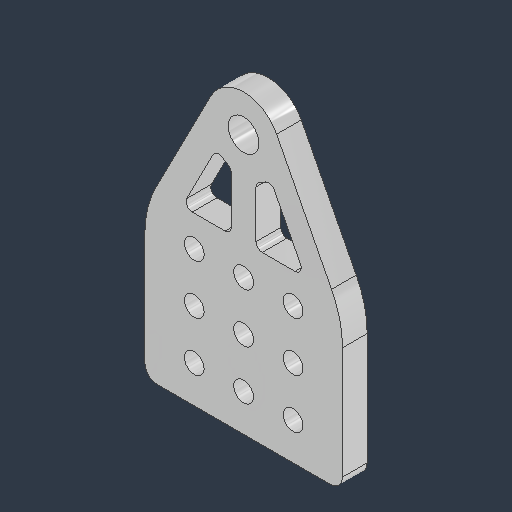
# Autodesk Inventor part: PLATE,SIDE,PULLEY,MOUNT,TOP,ELEVATORR
Saved by Autodesk Inventor 2024.3 (Build 283343000, 343)
## iProperties
ILogicPurgeVersion: 0.0.0.0
OnSaveVersion: 3.4.3.0
OnSaveAssembly: COREAutomationManager
Created: 2025-01-27
Part Number: PLATE,SIDE,PULLEY,MOUNT,TOP,ELEVATORR
Material: Aluminum 7075
Document SubType Name: Modeling
Designer: Jthib
Density: 2.81 g/cm^3
Appearance: Aluminum - Polished
Mfg Approved By: John.Thibert
Sheet Metal Rule: Default
Mass: 83.4067 g
Surface Area: 97.3008 cm^2
Volume: 29.6821 cm^3
ModelCat: Uncategorized
MaterialName: Aluminum 7075
CN_MASS: 0.08
Author: Jthib
Autodesk Inventor part; units mm, degrees
ref_plane "YZ Plane" through (0, 0, 0) normal (1, 0, 0) x (0, 1, 0)
ref_plane "XZ Plane" through (0, 0, 0) normal (0, 1, 0) x (-1, 0, 0)
ref_plane "XY Plane" through (0, 0, 0) normal (0, 0, 1) x (1, 0, 0)
sketch "Sketch1" plane through (0, 0, 0) normal (0, 0, 1) x (1, 0, 0)
  line L0 (25.4, 0) -> (-25.4, 0) construction
  line L1 (25.4, 0) -> (25.4, -38.1)
  line L2 (-25.4, -38.1) -> (-25.4, 0)
  line L3 (0, 57.7256) -> (0, -54.0709) construction
  line L4 (-25.4, -38.1) -> (25.4, -38.1)
  line L5 (25.4, 0) -> (8.4711, 32.9299)
  arc A0 (6.9296, 22.04) -> (3.175, 19.5947) centre (0, 28.575) ccw
  line L6 (-8.4711, 32.9299) -> (-25.4, 0)
  line L7 (15.8117, 4.7625) -> (6.9296, 22.04)
  line L8 (3.175, 19.5947) -> (3.175, 4.7625)
  line L9 (3.175, 4.7625) -> (15.8117, 4.7625)
  arc A1 (3.175, 19.5947) -> (6.9296, 22.04) centre (0, 28.575) ccw
  line L10 (-15.8117, 4.7625) -> (-6.9296, 22.04)
  line L11 (-3.175, 19.5947) -> (-3.175, 4.7625)
  line L12 (-3.175, 4.7625) -> (-15.8117, 4.7625)
  arc A2 (-6.9296, 22.04) -> (-3.175, 19.5947) centre (0, 28.575) ccw
  point P0 (0, 0)
  point P1 (0, 0)
  point P2 (-3.175, 19.5947)
  point P3 (-6.9296, 22.04)
  dimension "d112" = 28.575
  dimension "d113" = 9.525
  dimension "d114" = 50.8
  dimension "d115" = 38.1
  dimension "d117" = 6.35
  dimension "d118" = 4.7625
  dimension "d119" = 6.35
  constraints: 24 end point, 8 point on circle, 4 symmetric about line, 3 centre point, 3 parallel, 2 horizontal, 2 tangent, 2 vertical, 1 coincident, 1 midpoint, 1 perpendicular, 1 point on line, 2 other
  measures "d112" distance from line of L0 A0.centre
  measures "d113" radius of A0
  measures "d114" distance of L2.start L1.end
  measures "d115" distance of L0.start L1.end
  measures "d117" distance between parallel lines of L5 L7
  measures "d118" distance between parallel lines of L0 L9
  measures "d119" diameter of L8 L3
extrude "Extrusion2" add sketch "Sketch1" along normal mid plane 6.35 contours L1 L4 L2 L6 A0 L10 L12 L11 L8 L9 L7 L5 | A0 A1
sketch "Sketch3" plane through (0, 0, -3.175) normal (0, 0, -1) x (-1, 0, 0)
  line L0 (-35.56, 0) -> (35.56, 0) construction
  line L1 (0, -53.34) -> (0, 53.34) construction
  line L2 (12.7, -3.175) -> (-12.7, -3.175) construction
  line L3 (12.7, -15.875) -> (-12.7, -15.875) construction
  line L4 (12.7, -28.575) -> (-12.7, -28.575) construction
  point P0 (0, 0)
  point P1 (0, -3.175)
  point P2 (0, -15.875)
  point P3 (0, -28.575)
  dimension "d43" = 25.4
  dimension "d45" = 3.175
  dimension "d107" = 12.7
  constraints: 6 end point, 2 coincident, 1 horizontal, 1 midpoint, 1 point on line, 1 vertical, 8 other
  measures "d43" distance of L2.start L2.end
  measures "d45" distance between parallel lines of L0 L2
  measures "d107" distance of L2.start L3.start
hole "Hole2" at (12.7, -3.175, -3.175) at (-12.7, -3.175, -3.175) at (0, -3.175, -3.175) at (12.7, -15.875, -3.175) at (0, -15.875, -3.175) at (-12.7, -15.875, -3.175) at (12.7, -28.575, -3.175) at (0, -28.575, -3.175) at (-12.7, -28.575, -3.175) direction (0, 0, 1) diameter 5.1054 end through all clearance for "Flat Head Machine Screw (82)" size "#10" standard "Ansi Unified Screw Threads"
sketch "Sketch7" plane through (0, 0, -3.175) normal (0, 0, 1) x (1, 0, 0)
  arc A0 (8.4711, 32.9299) -> (-8.4711, 32.9299) centre (0, 28.575) ccw construction
  point P0 (0, 0)
  constraints: 1 coincident
hole "Hole4" at (0, 28.575, -3.175) direction (0, 0, 1) diameter 7.9375 end through all
fillet "Fillet5" radius 3.175 2 edges at (-25.4, -38.1, 0) (25.4, -38.1, 0)
fillet "Fillet7" radius 1.5875 8 edges at (-15.8117, 4.7625, 0) (-6.9296, 22.04, 0) (-3.175, 19.5947, 0) (-3.175, 4.7625, 0) (3.175, 4.7625, 0) (3.175, 19.5947, 0) (6.9296, 22.04, 0) (15.8117, 4.7625, 0)
fillet "Fillet9" radius 25.4 2 edges at (25.4, 0, 0) (-25.4, 0, 0)
equation "\"BendRadius\" = Thickness"
equation "\"BendReliefWidth\" = Thickness"
equation "\"BendReliefDepth\" = 0.5 * Thickness"
equation "\"CornerReliefSize\" = 4 * Thickness"
equation "\"MinimumRemnant\" = 2 * Thickness"
equation "\"TransitionRadius\" = BendRadius"
equation "\"JacobiRadiusSize\" = BendRadius"
equation "\"GapSize\" = Thickness"
equation "\"Thickness\" = 6.35"
body "Solid3"
